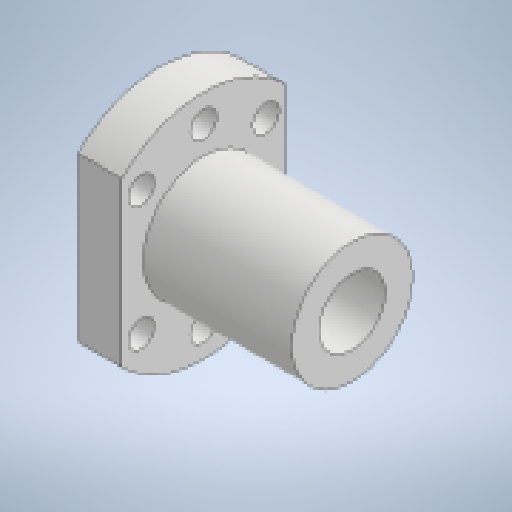
# Autodesk Inventor part: SFU1204-Housing
Saved by Autodesk Inventor 2023 (Build 270158000, 158)
## iProperties
Created: 2022-04-29
Part Number: SFU1204-Housing
Material: Generic
Document SubType Name: Modeling
Designer: plebbb
Density: 1 g/cm^3
Appearance: Default
Mass: 12.7251 g
Surface Area: 65.6682 cm^2
Volume: 12.7251 cm^3
Author: plebbb
Autodesk Inventor part; units mm, degrees
ref_plane "YZ Plane" through (0, 0, 0) normal (1, 0, 0) x (0, 1, 0)
ref_plane "XZ Plane" through (0, 0, 0) normal (0, 1, 0) x (-1, 0, 0)
ref_plane "XY Plane" through (0, 0, 0) normal (0, 0, 1) x (1, 0, 0)
sketch "Sketch1" plane through (0, 0, 0) normal (0, 0, 1) x (1, 0, 0)
  line L0 (0, 21) -> (0, 6)
  line L1 (0, 0) -> (35, 0) construction
  line L2 (35, 0) -> (35, 6) construction
  line L3 (35, 11) -> (8, 11)
  line L4 (8, 11) -> (8, 21)
  line L5 (8, 21) -> (0, 21)
  line L6 (35, 6) -> (0, 6)
  line L7 (0, 6) -> (0, 0) construction
  line L8 (35, 6) -> (35, 11)
  dimension "d0" = 11
  dimension "d1" = 21
  dimension "d2" = 8
  dimension "d3" = 35
  dimension "d4" = 6
  constraints: 18 end point, 8 perpendicular, 2 vertical, 1 coincident, 1 horizontal
  measures "d0" distance of L1.end L3.start
  measures "d1" distance of L0.start L1.start
  measures "d2" distance of L4.end L0.start
  measures "d3" horizontal distance of L3.start L0.start
  measures "d4" distance from line of point (0, 0) L6
revolve "Revolution1" add sketch "Sketch1" angle 360 about axis through (0, 0, 0) along (1, 0, 0)
sketch "Sketch2" plane through (0, 0, 0) normal (-1, 0, 0) x (0, 0, 1)
  circle A0 centre (0, 0) radius 21 projected
  circle A1 centre (0, 0) radius 21 projected
  line L0 (-14.8492, 14.8492) -> (-14.8492, -14.8492)
  line L1 (14.8492, -14.8492) -> (14.8492, 14.8492)
  line L2 (0, 0) -> (14.8492, 14.8492) construction
  circle A2 centre (0, 16) radius 2.4
  circle A3 centre (11.3137, 11.3137) radius 2.4
  circle A4 centre (11.3137, -11.3137) radius 2.4
  circle A5 centre (0, 0) radius 16 construction
  circle A6 centre (-11.3137, 11.3137) radius 2.4
  circle A7 centre (0, -16) radius 2.4
  circle A8 centre (-11.3137, -11.3137) radius 2.4
  point P0 (-14.8492, -14.8492)
  dimension "d6" = 45
  dimension "d7" = 32
  dimension "d8" = 4.8
  constraints: 10 point on circle, 7 centre point, 6 end point, 5 equal radius, 4 vertical alignment, 3 horizontal alignment, 2 parallel, 2 point on line, 1 coincident
  measures "d6" angle of L1 L2
  measures "d7" diameter of A5
  measures "d8" diameter of A2
extrude "Extrusion1" cut sketch "Sketch2" against normal blind 10 contours A0 L1 | L0 A0 | A2 | A3 | A4 | A6 | A7 | A8
body "Solid1"
